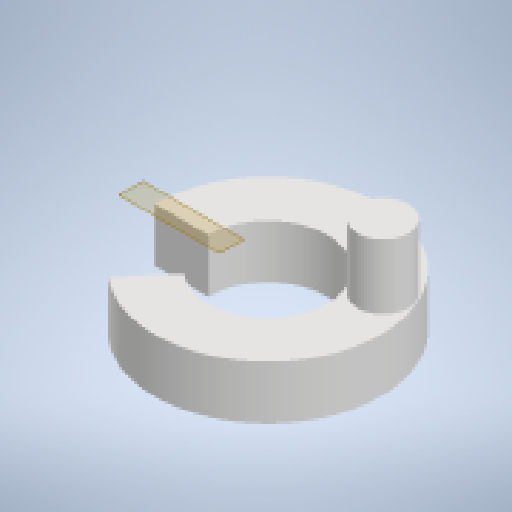
# Autodesk Inventor part: wash_ring
Saved by Autodesk Inventor 2023.3 (Build 273359000, 359)
## iProperties
Created: 2023-11-29
Part Number: wash_ring
Material: Generic
Document SubType Name: Modeling
Designer: mmelin
Density: 1 g/cm^3
Appearance: Default
Author: mmelin
Autodesk Inventor part; units mm, degrees
ref_plane "YZ Plane" through (0, 0, 0) normal (1, 0, 0) x (0, 1, 0)
ref_plane "XZ Plane" through (0, 0, 0) normal (0, 1, 0) x (-1, 0, 0)
ref_plane "XY Plane" through (0, 0, 0) normal (0, 0, 1) x (1, 0, 0)
sketch "Sketch1" plane through (0, 0, 0) normal (0, 0, 1) x (1, 0, 0)
  line L0 (20, 10.9474) -> (20, -17.8312)
  line L1 (-6.604, 6.604) -> (-6.604, -6.604) projected
  line L2 (-6.604, -6.604) -> (6.604, -6.604) projected
  line L3 (6.604, 6.604) -> (-6.604, 6.604) projected
  line L4 (6.604, -6.604) -> (6.604, 6.604) projected
  line L5 (-6.204, -6.204) -> (6.204, -6.204)
  line L6 (6.204, -6.204) -> (6.204, 6.204)
  line L7 (6.204, 6.204) -> (-6.204, 6.204)
  line L8 (-6.204, 6.204) -> (-6.204, -6.204)
  point P0 (0, 0)
  dimension "d2" = 20
  dimension "d8" = 0.4
  dimension "d9" = 0.4
  dimension "d10" = 0.4
  dimension "d11" = 0.4
  constraints: 10 end point, 2 parallel, 1 horizontal, 1 perpendicular, 1 vertical
  measures "d2" distance from line of L0 point (0, 0)
  measures "d8" distance between parallel lines of L1 L8
  measures "d9" distance between parallel lines of L3 L7
  measures "d10" distance between parallel lines of L4 L6
  measures "d11" distance between parallel lines of L2 L5
revolve "Revolution1" add sketch "Sketch1" angle 310 about axis through (20, 10.9474, 0) along (0, -1, 0) contours L8 L7 L6 L5
ref_plane "Work Plane1" through (0, 6.604, 2.5) normal (0, 1, 0) x (0, 0, 1)
sketch "Sketch4" plane through (-6.204, 6.204, 0) normal (0, 1, 0) x (1, 0, 0)
  line L0 (0, 0) -> (12.408, 0) projected
  line L1 (0, 0) -> (52.408, 0) construction
  arc A0 (9.3604, -20.0734) -> (0, 0) centre (26.204, 0) ccw projected
  line L2 (9.3604, -20.0734) -> (43.0476, 20.0734) construction
  line L3 (9.3604, -20.0734) -> (17.3361, -10.5683) construction
  line L4 (12.408, 0) -> (0, 0) construction
  circle A1 centre (44.2932, 8.4352) radius 5.904
  line L5 (44.2932, 8.4352) -> (43.0476, 20.0734)
  line L6 (44.2932, 8.4352) -> (52.408, 0)
  point P0 (6.204, 0)
  dimension "d15" = 11.808
  dimension "d16" = 8.4352
  constraints: 8 end point, 2 collinear, 2 point on circle, 1 centre point, 1 equal length
  measures "d15" diameter of A1
  measures "d16" vertical distance of L5.start L1.end
extrude "Extrusion3" add sketch "Sketch4" along normal blind 15 contours L6 L5 A1 | A1 L5 L6
equation "\"d9\" = d8"
equation "\"d10\" = d8"
equation "\"d11\" = d8"
body "Solid1"
